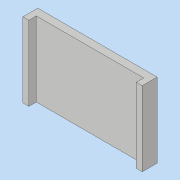
# Autodesk Inventor part: USBBreakoutCover
Saved by Autodesk Inventor 2017 (Build 210142000, 142)
## iProperties
Created: 2019-07-16
Part Number: USBBreakoutCover
Material: Generic
Document SubType Name: Modeling
Designer: techn
Density: 1 g/cm^3
Appearance: Default
Author: techn
Autodesk Inventor part; units mm, degrees
ref_plane "YZ Plane" through (0, 0, 0) normal (1, 0, 0) x (0, 1, 0)
ref_plane "XZ Plane" through (0, 0, 0) normal (0, 1, 0) x (-1, 0, 0)
ref_plane "XY Plane" through (0, 0, 0) normal (0, 0, 1) x (1, 0, 0)
sketch "Sketch1" plane through (0, 0, 0) normal (0, 0, 1) x (1, 0, 0)
  line L0 (0, 0) -> (20.32, 0)
  line L1 (20.32, 0) -> (20.32, 12.7)
  line L2 (20.32, 12.7) -> (0, 12.7)
  line L3 (0, 12.7) -> (0, 0)
  dimension "d0" = 20.32
  dimension "d1" = 12.7
  constraints: 8 end point, 2 parallel, 1 horizontal, 1 perpendicular
  measures "d0" distance of L1.end L2.end
  measures "d1" distance of L0.end L1.end
extrude "Extrusion1" add sketch "Sketch1" along normal blind 1.27
sketch "Sketch2" plane through (0, 0, 1.27) normal (0, 0, 1) x (1, 0, 0)
  line L0 (20.32, 12.7) -> (0, 12.7) projected
  line L1 (0, 0) -> (1.016, 0)
  line L2 (1.016, 0) -> (1.016, 12.7)
  line L3 (1.016, 12.7) -> (0, 12.7)
  line L4 (0, 12.7) -> (0, 0)
  line L5 (20.32, 12.7) -> (19.304, 12.7)
  line L6 (19.304, 12.7) -> (19.304, 0)
  line L7 (19.304, 0) -> (20.32, 0)
  line L8 (20.32, 0) -> (20.32, 12.7)
  dimension "d4" = 1.016
  dimension "d5" = 1.016
  constraints: 16 end point, 4 parallel, 2 horizontal, 2 perpendicular, 2 point on line
  measures "d4" distance between parallel lines of L4 L2
  measures "d5" distance between parallel lines of L8 L6
extrude "Extrusion2" add sketch "Sketch2" along normal blind 1.27
body "Solid1"
